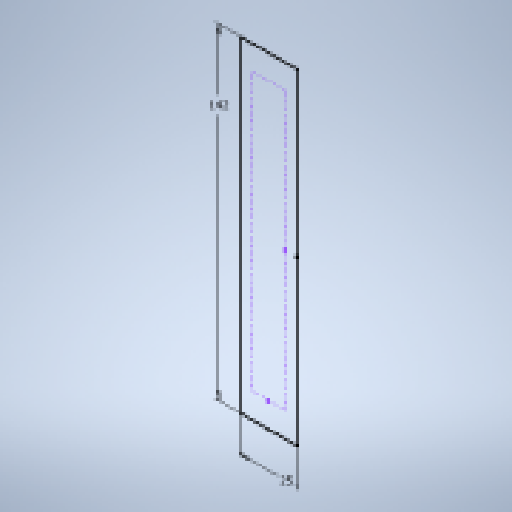
# Autodesk Inventor part: Watercooler_Mounting_Plate
Saved by Autodesk Inventor 2023 (Build 270158000, 158)
## iProperties
Created: 2023-08-19
Part Number: Watercooler_Mounting_Plate
Material: Generic
Document SubType Name: Modeling
Designer: plebbb
Density: 1 g/cm^3
Appearance: Default
Author: plebbb
Autodesk Inventor part; units mm, degrees
ref_plane "YZ Plane" through (0, 0, 0) normal (1, 0, 0) x (0, 1, 0)
ref_plane "XZ Plane" through (0, 0, 0) normal (0, 1, 0) x (-1, 0, 0)
ref_plane "XY Plane" through (0, 0, 0) normal (0, 0, 1) x (1, 0, 0)
sketch "Sketch1" plane through (0, 0, 0) normal (0, 0, 1) x (1, 0, 0)
  line L0 (0, 0) -> (25, 0)
  line L1 (25, 0) -> (25, -142)
  line L2 (25, -142) -> (0, -142)
  line L3 (0, -142) -> (0, 0)
  line L4 (20, -5.35) -> (5, -5.35) construction
  line L5 (5, -5.35) -> (5, -136.65) construction
  line L6 (5, -136.65) -> (20, -136.65) construction
  line L7 (20, -136.65) -> (20, -5.35) construction
  circle A0 centre (20, -5.35) radius 2.794
  circle A1 centre (5, -5.35) radius 2.794
  circle A2 centre (20, -136.65) radius 2.794
  circle A3 centre (5, -136.65) radius 2.794
  line L8 (0, 0) -> (-24, 0)
  line L9 (-24, 0) -> (-24, -142)
  line L10 (-24, -142) -> (0, -142)
  line L11 (25, -142) -> (37, -142)
  line L12 (37, -142) -> (37, 0)
  line L13 (37, 0) -> (25, 0)
  point P0 (20, -71)
  point P1 (25, -71)
  point P2 (12.5, -136.65)
  point P3 (12.5, -142)
  dimension "d0" = 142
  dimension "d1" = 25
  dimension "d2" = 131.3
  dimension "d3" = 15
  dimension "d4" = 5.588
  dimension "d7" = 12
  dimension "d8" = 24
  constraints: 28 end point, 5 perpendicular, 4 centre point, 4 coincident, 4 midpoint, 4 parallel, 3 equal radius, 3 horizontal, 3 point on line, 1 collinear, 1 horizontal alignment, 1 vertical alignment
  measures "d0" distance of L2.end L0.start
  measures "d1" distance of L1.end L2.end
  measures "d2" distance of L6.end L4.start
  measures "d3" distance of L5.end L6.end
  measures "d4" diameter of A0
  measures "d7" distance of L12.end L0.end
  measures "d8" distance of L0.start L8.end
extrude "Extrusion1" add sketch "Sketch1" along normal blind 3
sketch "Sketch2" plane through (0, 0, 3) normal (0, 0, 1) x (1, 0, 0)
  line L0 (26.3967, -88.79) -> (-13.3967, -88.79) construction
  line L1 (-13.3967, -88.79) -> (-13.3967, -60.85) construction
  line L2 (-13.3967, -60.85) -> (26.3967, -60.85) construction
  line L3 (26.3967, -60.85) -> (26.3967, -88.79) construction
  line L4 (-24, -142) -> (37, -142) construction
  circle A0 centre (26.3967, -60.85) radius 2.0828
  circle A1 centre (26.3967, -88.79) radius 2.0828
  circle A2 centre (-13.3967, -60.85) radius 2.0828
  circle A3 centre (-13.3967, -88.79) radius 2.0828
  point P0 (0, 0)
  point P1 (6.5, -88.79)
  point P2 (6.5, -142)
  dimension "d9" = 53.21
  dimension "d10" = 27.94
  dimension "d11" = 39.7933
  dimension "d12" = 4.1656
  constraints: 8 end point, 4 centre point, 4 coincident, 3 equal radius, 2 midpoint, 2 parallel, 1 horizontal, 1 perpendicular, 1 vertical alignment
  measures "d9" distance between parallel lines of L4 L0
  measures "d10" distance of L0.end L1.end
  measures "d11" distance of L0.start L0.end
  measures "d12" diameter of A0
extrude "Extrusion2" cut sketch "Sketch2" against normal blind 3
body "Solid1"
